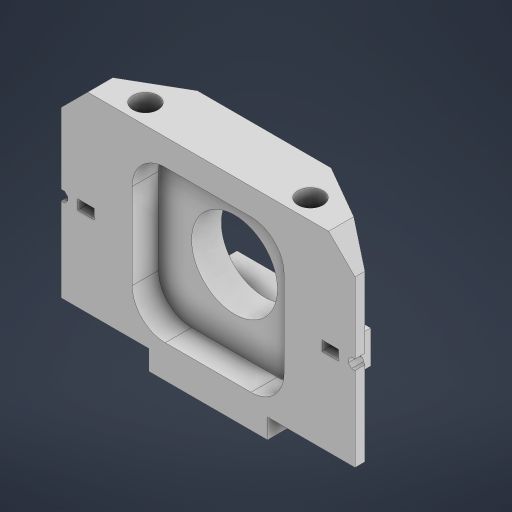
# Autodesk Inventor part: Endkappe plus Federhalter 3D
Saved by Autodesk Inventor 2024.2 (Build 282272000, 272)
## iProperties
Created: 2024-04-01
Part Number: Endkappe plus Federhalter 3D
Material: Generisch
Document SubType Name: Modeling
Designer: luhsoccer
Density: 1 g/cm^3
Appearance: Vorgabe
Author: luhsoccer
## iProperties of the stored document Endkappe plus Federhalter 3D_3D-Druck.ipt
Created: 2024-04-01
Part Number: Endkappe plus Federhalter 3D_3D-Druck
Material: Generisch
Document SubType Name: Modeling
Designer: luhsoccer
Density: 1 g/cm^3
Appearance: Vorgabe
Author: luhsoccer
Autodesk Inventor part; units mm, degrees
ref_plane "YZ Plane" through (0, 0, 0) normal (1, 0, 0) x (0, 1, 0)
ref_plane "XZ Plane" through (0, 0, 0) normal (0, 1, 0) x (-1, 0, 0)
ref_plane "XY Plane" through (0, 0, 0) normal (0, 0, 1) x (1, 0, 0)
sketch "Skizze1" plane through (0, 0, 0) normal (0, 1, 0) x (-1, 0, 0)
  circle A0 centre (0, 0) radius 6.5
  line L0 (9, -16.5) -> (-9, -16.5)
  line L1 (-9, -16.5) -> (-9, -13.5)
  line L2 (-9, -16.5) -> (-6, -16.5) construction
  line L3 (9, -16.5) -> (9, -13.5)
  line L4 (9, -16.5) -> (12, -16.5) construction
  line L5 (22.25, -13.5) -> (-22.25, -13.5)
  line L6 (22.25, -13.5) -> (22.25, 15.5)
  line L7 (22.25, 15.5) -> (-22.25, 15.5)
  line L8 (-22.25, 15.5) -> (-22.25, -13.5)
  line L9 (6.5, 11.5) -> (-6.5, 11.5)
  line L10 (-11.5, 6.5) -> (-11.5, -6.5)
  line L11 (-6.5, -11.5) -> (6.5, -11.5)
  line L12 (11.5, -6.5) -> (11.5, 6.5)
  arc A1 (11.5, 6.5) -> (6.5, 11.5) centre (6.5, 6.5) ccw
  arc A2 (-6.5, 11.5) -> (-11.5, 6.5) centre (-6.5, 6.5) ccw
  arc A3 (-11.5, -6.5) -> (-6.5, -11.5) centre (-6.5, -6.5) ccw
  arc A4 (6.5, -11.5) -> (11.5, -6.5) centre (6.5, -6.5) ccw
  point P0 (0, -16.5)
  point P1 (0, 11.5)
  point P2 (0, 15.5)
  point P3 (11.5, 11.5)
  point P4 (-11.5, -11.5)
  point P5 (-11.5, 11.5)
  point P6 (11.5, -11.5)
  point P7 (0, 11.5)
  point P8 (-11.5, 0)
  point P9 (-9, -13.5)
  point P10 (9, -13.5)
  dimension "d0" = 13
  dimension "d1" = 18
  dimension "d2" = 3
  dimension "d3" = 90
  dimension "d4" = 3
  dimension "d5" = 90
  dimension "d6" = 44.5
  dimension "d7" = 13.25
  dimension "d8" = 29
  dimension "d15" = 23
  dimension "d16" = 23
  dimension "d17" = 4
  dimension "d18" = 5
  dimension "d23" = 5
  constraints: 26 end point, 8 point on circle, 8 point on line, 8 tangent, 5 centre point, 5 horizontal, 5 perpendicular, 4 midpoint, 3 equal radius, 3 vertical, 3 vertical alignment, 2 parallel, 1 coincident, 1 horizontal alignment
  measures "d0" diameter of A0
  measures "d1" distance of L0.start L0.end
  measures "d2" distance of L0.end L1.end
  measures "d3" angle of L2 L1
  measures "d4" distance of L0.start L3.end
  measures "d5" angle of L4 L3
  measures "d6" distance of L5.start L5.end
  measures "d7" distance from line of L1 L5.end
  measures "d8" distance of L5.start L6.end
  measures "d15" distance of point (11.5, -11.5) point (-11.5, -11.5)
  measures "d16" distance of point (-11.5, -11.5) point (-11.5, 11.5)
  measures "d17" distance between parallel lines of L7 L9
  measures "d18" distance between parallel lines of L11 L0
  measures "d23" radius of A1
extrude "Extrusion1" add sketch "Skizze1" along normal blind 8.5 contours L0 L1 L5 L3 | L5 L8 L7 L6 | A1 L12 A4 L11 A3 L10 A2 L9
extrude "Extrusion2" cut sketch "Skizze1" along normal blind 4 contours A1 L12 A4 L11 A3 L10 A2 L9
sketch "Skizze Bohrung inserts" plane through (-9, 0, -13.5) normal (0, 0, -1) x (-1, 0, 0)
  line L0 (4.9, 3) -> (-22.9, 3)
  line L1 (2.5, 0) -> (-2.5, 0) projected
  point P0 (-9, 0)
  point P1 (-9, 3)
  dimension "d24" = 27.8
  dimension "d25" = 3
  constraints: 2 end point, 1 horizontal, 1 midpoint, 1 vertical alignment
  measures "d24" distance of L0.start L0.end
  measures "d25" distance between parallel lines of L1 L0
hole "Bohrung1" at (-13.9, 3, -13.5) at (13.9, 3, -13.5) direction (0, 0, 1) diameter 3.8 depth 6.8 tip angle 118
chamfer "Fasen1" distance 4 angle 45 2 edges at (-22.25, 4.25, 15.5) (22.25, 4.25, 15.5)
sketch "Skizze3" plane through (9, 0, -16.5) normal (0, 0, -1) x (-1, 0, 0)
  line L0 (0, 0) -> (18, 0) projected
  line L1 (18, 0) -> (18, 8.5) projected
  line L2 (0, 8.5) -> (18, 8.5) projected
  line L3 (0, 0) -> (0, 8.5) projected
  line L4 (0, 8.5) -> (18, 8.5) projected
  line L5 (0, 8.5) -> (18, 8.5)
  line L6 (18, 8.5) -> (18, 6)
  line L7 (18, 6) -> (0, 6)
  line L8 (0, 6) -> (0, 8.5)
  point P0 (9, 0)
  point P1 (0, 6)
  dimension "d36" = 6
  constraints: 8 end point, 2 parallel, 1 horizontal, 1 perpendicular, 1 point on line
  measures "d36" distance between parallel lines of L0 L7
extrude "Extrusion3" cut sketch "Skizze3" against normal up to surface (3 mm away) contours L3 L2 L1 L7
sketch "Skizze4" plane through (0, 0, 0) normal (0, -1, 0) x (1, 0, 0)
  line L0 (-19.75, 0.75) -> (-17.25, 0.75)
  line L1 (-17.25, 0.75) -> (-17.25, -0.75)
  line L2 (-17.25, -0.75) -> (-19.75, -0.75)
  line L3 (-19.75, -0.75) -> (-19.75, 0.75)
  line L4 (-22.25, -13.5) -> (-22.25, 11.5) projected
  point P0 (0, 0)
  point P1 (-17.25, 0)
  dimension "d39" = 2.5
  dimension "d40" = 1.5
  dimension "d41" = 2.5
  constraints: 8 end point, 2 parallel, 1 horizontal, 1 horizontal alignment, 1 midpoint, 1 perpendicular
  measures "d39" distance of L1.end L2.end
  measures "d40" distance of L0.end L1.end
  measures "d41" distance between parallel lines of L3 L4
extrude "Extrusion4" cut sketch "Skizze4" against normal blind 5
sketch "Skizze5" plane through (-19.75, 0, 0.75) normal (1, 0, 0) x (0, 0, -1)
  line L0 (1.5, 0) -> (0, 0) projected
  line L1 (1.5, 0) -> (1.5, 5) projected
  line L2 (1.5, 5) -> (0, 5) projected
  line L3 (0, 0) -> (0, 5) projected
  line L4 (0, 0) -> (0, 1)
  line L5 (0, 1) -> (1.25, 1)
  line L6 (1.25, 1) -> (0, 2.25)
  line L7 (0.25, 1) -> (1.5, 2.25)
  line L8 (0.25, 1) -> (2.0178, 1) construction
  line L9 (1.5, 2.25) -> (1.5, 5)
  line L10 (0, 2.25) -> (0, 5)
  line L11 (1.5, 5) -> (0, 5)
  point P0 (0.75, 0)
  point P1 (0.75, 1.5)
  dimension "d44" = 1
  dimension "d45" = 45
  dimension "d46" = 45
  constraints: 16 end point, 3 point on line, 2 collinear, 1 equal length, 1 horizontal, 1 perpendicular, 1 vertical
  measures "d44" distance of L0.end L4.end
  measures "d45" angle of L6 L5
  measures "d46" angle of L8 L7
extrude "Extrusion5" cut sketch "Skizze5" against normal up to surface (2.5 mm away) contours L7 L6 L3 L2 L1
sketch "Skizze7" plane through (-22.25, 0, -13.5) normal (-1, 0, 0) x (0, 0, 1)
  line L0 (13.5, 1.5) -> (14.25, 2.25) projected
  line L1 (14.25, 2.25) -> (14.25, 0)
  line L2 (20, 0) -> (7, 0) projected
  line L3 (12.75, 2.25) -> (13.5, 1.5) projected
  line L4 (12.75, 2.25) -> (12.75, 0)
  line L5 (12.75, 0) -> (14.25, 0)
  line L6 (13.5, 1.5) -> (12.75, 2.25) projected
  line L7 (14.25, 2.25) -> (13.5, 1.5) projected
  line L8 (13.5, 1.5) -> (14.25, 2.25)
  line L9 (13.5, 1.5) -> (12.75, 2.25)
  point P0 (13.5, 0)
  constraints: 10 end point, 2 vertical, 1 collinear, 1 perpendicular, 1 point on line
extrude "Extrusion7" cut sketch "Skizze7" against normal blind 1
mirror "Spiegeln1" about plane through (0, 0, 0) normal (1, 0, 0) of "Extrusion5", "Extrusion4", "Extrusion7"
chamfer "Fasen4" distance 0.75 angle 45 5 edges at (-19.75, 5, 0.75) (-19.75, 5, -0.75) (-17.25, 5, 0) (19.75, 5, -0.75) (19.75, 5, 0.75)
chamfer "Fasen5" distance 0.5 angle 45 4 edges at (-21.25, 1.125, 0.75) (-21.25, 1.125, -0.75) (21.25, 1.125, 0.75) (21.25, 1.125, -0.75)
chamfer "Fasen6" distance 7 angle 60 1 edges at (-22.25, 8.5, -1)
chamfer "Fasen7" distance 7 angle 60 1 edges at (22.25, 8.5, -1)
sketch "Skizze9" plane through (0, 8.5, 0) normal (0, 1, 0) x (1, 0, 0)
  line L0 (22.25, 13.5) -> (10.1256, 13.5) projected
  line L1 (-10.1256, -15.5) -> (-10.1256, 13.5) projected
  line L2 (10.1256, 13.5) -> (-10.1256, 13.5)
  line L3 (-10.1256, 13.5) -> (-10.1256, 8.5)
  line L4 (-10.1256, 8.5) -> (10.1256, 8.5)
  line L5 (10.1256, 8.5) -> (10.1256, 13.5)
  point P0 (0, 0)
  point P1 (13.322, 13.5)
  dimension "d76" = 5
  constraints: 8 end point, 2 parallel, 1 horizontal, 1 perpendicular, 1 point on line
  measures "d76" distance between parallel lines of L4 L2
extrude "Extrusion9" add sketch "Skizze9" along normal blind 6
sketch "Skizze10" plane through (-18.25, 0, 15.5) normal (0, 0, 1) x (1, 0, 0)
  circle A0 centre (4.35, 3) radius 1.9 projected
  circle A1 centre (32.15, 3) radius 1.9 projected
  point P0 (18.25, 0)
  point P1 (5.75, 3)
  point P2 (30.75, 3)
  dimension "d86" = 1.4
  dimension "d87" = 1.4
  constraints: 2 horizontal alignment
  measures "d86" distance of A1.centre point (30.75, 3)
  measures "d87" distance of A0.centre point (5.75, 3)
hole "Bohrung2" at (-12.5, 3, 15.5) at (12.5, 3, 15.5) direction (0, 0, -1) diameter 3.8 depth 5.8
